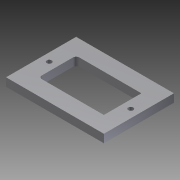
# Autodesk Inventor part: cetakan sepatu 3
Saved by Autodesk Inventor 2012 (Build 160160000, 160)
## iProperties
Created: 2014-01-20
Part Number: cetakan sepatu 3
Material: Default
Document SubType Name: Modeling
Designer: Irwan Haryanto
Density: 1 g/cm^3
Author: Irwan Haryanto
Autodesk Inventor part; units mm, degrees
ref_plane "YZ Plane" through (0, 0, 0) normal (1, 0, 0) x (0, 1, 0)
ref_plane "XZ Plane" through (0, 0, 0) normal (0, 1, 0) x (-1, 0, 0)
ref_plane "XY Plane" through (0, 0, 0) normal (0, 0, 1) x (1, 0, 0)
sketch "Sketch1" plane through (0, 0, 0) normal (0, 0, 1) x (1, 0, 0)
  circle A0 centre (-40.1802, -86.5414) radius 1.5
  line L0 (-35.1802, -108.0414) -> (-45.1802, -108.0414)
  line L1 (-35.1802, -65.0414) -> (-35.1802, -108.0414)
  line L2 (-45.1802, -65.0414) -> (-35.1802, -65.0414)
  line L3 (-45.1802, -98.0414) -> (-45.1802, -75.0414)
  line L4 (-83.1802, -98.0414) -> (-45.1802, -98.0414)
  line L5 (-45.1802, -75.0414) -> (-83.1802, -75.0414)
  line L6 (-45.1802, -65.0414) -> (-95.1802, -65.0414)
  line L7 (-95.1802, -108.0414) -> (-45.1802, -108.0414)
  arc A1 (-85.1802, -96.0414) -> (-83.1802, -98.0414) centre (-83.1802, -96.0414) ccw
  arc A2 (-83.1802, -75.0414) -> (-85.1802, -77.0414) centre (-83.1802, -77.0414) ccw
  line L8 (-85.1802, -77.0414) -> (-85.1802, -96.0414)
  circle A3 centre (-90.1802, -86.5414) radius 1.5
  line L9 (-95.1802, -65.0414) -> (-95.1802, -108.0414)
  point P0 (0, 0)
  dimension "d0" = 2
  dimension "d1" = 43
  dimension "d2" = 3
  dimension "d3" = 5
  dimension "d4" = 21.5
  dimension "d5" = 3
  dimension "d6" = 5
  dimension "d7" = 21.5
  constraints: 20 end point, 4 centre point, 4 perpendicular, 4 point on circle, 4 tangent, 3 parallel, 1 equal radius
  measures "d0" radius of A2
  measures "d1" distance of L6.end L7.start
  measures "d2" diameter of A3
  measures "d3" distance from line of A3.centre L9
  measures "d4" distance from line of L6 A3.centre
  measures "d5" diameter of A0
  measures "d6" distance from line of L1 A0.centre
  measures "d7" distance from line of L2 A0.centre
extrude "Extrusion1" add sketch "Sketch1" along normal blind 5
body "Solid1"
